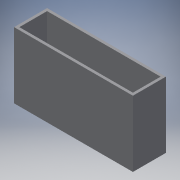
# Autodesk Inventor part: Bevel holder
Saved by Autodesk Inventor 2019 (Build 230136000, 136)
## iProperties
Created: 2019-10-27
Part Number: Bevel holder
Material: Generic
Document SubType Name: Modeling
Designer: Mark
Density: 1 g/cm^3
Appearance: Default
Author: Mark
Autodesk Inventor part; units mm, degrees
ref_plane "YZ Plane" through (0, 0, 0) normal (1, 0, 0) x (0, 1, 0)
ref_plane "XZ Plane" through (0, 0, 0) normal (0, 1, 0) x (-1, 0, 0)
ref_plane "XY Plane" through (0, 0, 0) normal (0, 0, 1) x (1, 0, 0)
sketch "Sketch1" plane through (0, 0, 0) normal (0, 1, 0) x (-1, 0, 0)
  line L0 (45, 12.5) -> (-45, 12.5)
  line L1 (-45, 12.5) -> (-45, -12.5)
  line L2 (-45, -12.5) -> (45, -12.5)
  line L3 (45, -12.5) -> (45, 12.5)
  line L4 (45, 12.5) -> (-45, -12.5) construction
  line L5 (-45, 12.5) -> (45, -12.5) construction
  line L6 (43, 10.5) -> (-43, 10.5)
  line L7 (-43, 10.5) -> (-43, -10.5)
  line L8 (-43, -10.5) -> (43, -10.5)
  line L9 (43, -10.5) -> (43, 10.5)
  line L10 (43, 10.5) -> (-43, -10.5) construction
  line L11 (-43, 10.5) -> (43, -10.5) construction
  point P0 (0, 0)
  dimension "d0" = 90
  dimension "d1" = 25
  dimension "d2" = 86
  dimension "d3" = 21
  constraints: 24 end point, 4 midpoint, 4 parallel, 2 horizontal, 2 perpendicular
  measures "d0" distance of L2.end L1.end
  measures "d1" distance of L1.end L0.end
  measures "d2" distance of L8.end L7.end
  measures "d3" distance of L7.end L6.end
extrude "Extrusion1" add sketch "Sketch1" along normal blind 50
body "Solid1"
